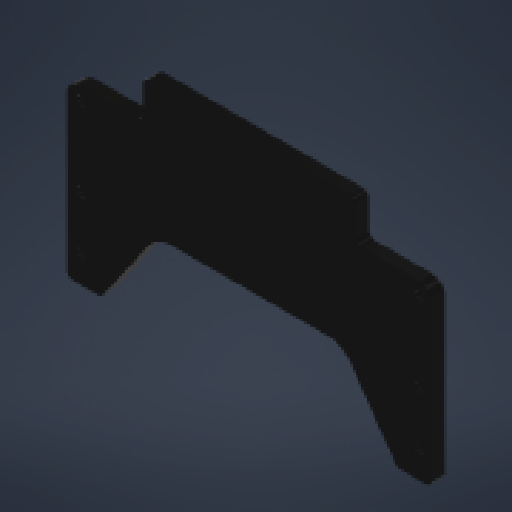
# Autodesk Inventor part: backalignermidgoal
Saved by Autodesk Inventor 2025.2 (Build 292293000, 293)
## iProperties
Created: 2026-01-01
Part Number: backalignermidgoal
Material: Acetal Resin, Black
Document SubType Name: Modeling
Designer: cloudy
Density: 1.425 g/cm^3
Appearance: Smooth - Black
Author: cloudy
Autodesk Inventor part; units mm, degrees
ref_plane "YZ Plane" through (0, 0, 0) normal (1, 0, 0) x (0, 1, 0)
ref_plane "XZ Plane" through (0, 0, 0) normal (0, 1, 0) x (-1, 0, 0)
ref_plane "XY Plane" through (0, 0, 0) normal (0, 0, 1) x (1, 0, 0)
sketch "Sketch1" plane through (0, 0, 0) normal (0, 0, 1) x (1, 0, 0)
  circle A0 centre (12.7, -88.9) radius 2.1844 projected
  circle A1 centre (-149.225, -88.9) radius 2.1844 projected
  circle A2 centre (12.7, -25.4) radius 2.1844 projected
  circle A3 centre (-149.225, -25.4) radius 2.1844 projected
  circle A4 centre (-149.225, -63.5) radius 2.1844 projected
  circle A5 centre (12.7, -63.5) radius 2.1844 projected
  line L0 (12.7, -19.05) -> (-149.225, -19.05)
  line L1 (-155.575, -25.4) -> (-155.575, -98.425)
  line L2 (-152.4, -101.6) -> (-140.7239, -101.6)
  line L3 (-138.1125, -100.2308) -> (-116.4997, -68.9766)
  line L4 (-106.054, -63.5) -> (-30.471, -63.5)
  line L5 (-20.0253, -68.9766) -> (1.5875, -100.2308)
  line L6 (4.1989, -101.6) -> (15.875, -101.6)
  line L7 (19.05, -98.425) -> (19.05, -25.4)
  arc A6 (19.05, -25.4) -> (12.7, -19.05) centre (12.7, -25.4) ccw
  arc A7 (-149.225, -19.05) -> (-155.575, -25.4) centre (-149.225, -25.4) ccw
  arc A8 (15.875, -101.6) -> (19.05, -98.425) centre (15.875, -98.425) ccw
  arc A9 (1.5875, -100.2308) -> (4.1989, -101.6) centre (4.1989, -98.425) ccw
  arc A10 (-140.7239, -101.6) -> (-138.1125, -100.2308) centre (-140.7239, -98.425) ccw
  arc A11 (-155.575, -98.425) -> (-152.4, -101.6) centre (-152.4, -98.425) ccw
  line L8 (-68.2625, -19.05) -> (-68.2625, -63.5) construction
  arc A12 (-20.0253, -68.9766) -> (-30.471, -63.5) centre (-30.471, -76.2) ccw
  arc A13 (-106.054, -63.5) -> (-116.4997, -68.9766) centre (-106.054, -76.2) ccw
  line L9 (-119.0625, -19.05) -> (-119.0625, 0)
  line L10 (-119.0625, 0) -> (-17.4625, 0)
  line L11 (-17.4625, 0) -> (-17.4625, -19.05)
  point P0 (0, 0)
  point P1 (-112.7125, -63.5)
  point P2 (-23.8125, -63.5)
  dimension "d0" = 6.35
  dimension "d2" = 3.175
  dimension "d3" = 12.7
  dimension "d4" = 88.9
  dimension "d5" = 44.45
  dimension "d6" = 25.4
  dimension "d7" = 12.7
  dimension "d23" = 101.6
  dimension "d24" = 19.05
  constraints: 24 end point, 16 point on circle, 16 tangent, 8 centre point, 6 point on line, 5 perpendicular, 4 equal radius, 2 coincident, 2 midpoint, 2 parallel, 2 vertical, 1 collinear, 1 horizontal, 2 other
  measures "d0" radius of A6
  measures "d2" radius of A8
  measures "d3" distance from line of A1.centre L2
  measures "d4" distance of point (-112.712, -63.5) point (-23.812, -63.5)
  measures "d5" distance between parallel lines of L0 L4
  measures "d6" horizontal distance of point (-23.812, -63.5) L5.end
  measures "d7" radius of A12
  measures "d23" diameter of L9 L8
  measures "d24" distance between parallel lines of L0 L10
extrude "Extrusion1" add sketch "Sketch1" along normal blind 6.35
fillet "Fillet2" radius 3.175 4 edges at (-119.0625, 0, 3.175) (-119.0625, -19.05, 3.175) (-17.4625, 0, 3.175) (-17.4625, -19.05, 3.175)
sketch "Sketch3" plane through (0, 0, 6.35) normal (0, 0, 1) x (1, 0, 0)
  circle A0 centre (12.7, -25.4) radius 2.1844 projected
  circle A1 centre (12.7, -25.4) radius 4.7625
  circle A2 centre (12.7, -63.5) radius 2.1844 projected
  circle A3 centre (12.7, -63.5) radius 4.7625
  circle A4 centre (-149.225, -25.4) radius 2.1844 projected
  circle A5 centre (-149.225, -25.4) radius 4.7625
  circle A6 centre (-149.225, -63.5) radius 2.1844 projected
  circle A7 centre (-149.225, -63.5) radius 4.7625
  point P0 (0, 0)
  dimension "d26" = 9.525
  dimension "d27" = 9.525
  dimension "d28" = 9.525
  dimension "d29" = 9.525
  constraints: 4 centre point, 4 coincident
  measures "d26" diameter of A1
  measures "d27" diameter of A3
  measures "d28" diameter of A5
  measures "d29" diameter of A7
extrude "Extrusion3" cut sketch "Sketch3" against normal blind 3.175 contours A0 | A1 | A2 | A3 | A4 | A5 | A6 | A7
body "Solid1"
